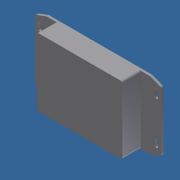
# Autodesk Inventor part: LIDAR PSU
Saved by Autodesk Inventor 2012 (Build 160160000, 160)
## iProperties
Created: 2012-03-25
Part Number: LIDAR PSU
Material: Default
Document SubType Name: Modeling
Designer: Edward
Mass: 374.214 g
Surface Area: 436.694 cm^2
Volume: 324.722 cm^3
Density: 1.15241 g/cm^3
Author: Edward
Autodesk Inventor part; units mm, degrees
ref_plane "YZ Plane" through (0, 0, 0) normal (1, 0, 0) x (0, 1, 0)
ref_plane "XZ Plane" through (0, 0, 0) normal (0, 1, 0) x (-1, 0, 0)
ref_plane "XY Plane" through (0, 0, 0) normal (0, 0, 1) x (1, 0, 0)
sketch "Sketch1" plane through (0, 0, 0) normal (0, 0, 1) x (1, 0, 0)
  line L0 (-7.8312, -44.5359) -> (133.0626, -44.5359)
  line L1 (133.0626, -44.5359) -> (133.0626, 47.9201)
  line L2 (133.0626, 47.9201) -> (-7.8312, 47.9201)
  line L3 (-7.8312, 47.9201) -> (-7.8312, -44.5359)
  line L4 (-7.8312, 47.9201) -> (-21.6516, 42.767)
  arc A0 (-21.6516, 42.767) -> (-23.7173, 39.7921) centre (-20.5423, 39.7921) ccw
  line L5 (-23.7173, 39.7921) -> (-23.7173, -36.4079)
  arc A1 (-23.7173, -36.4079) -> (-21.6516, -39.3828) centre (-20.5423, -36.4079) ccw
  line L6 (-21.6516, -39.3828) -> (-7.8312, -44.5359)
  circle A2 centre (-17.0085, 33.8104) radius 2.1971
  circle A3 centre (-17.0085, 27.689) radius 2.1971
  line L7 (-19.2056, 33.8104) -> (-14.8114, 33.8104)
  line L8 (-14.8114, 33.8104) -> (-14.8114, 27.689)
  line L9 (-14.8114, 27.689) -> (-19.2056, 27.689)
  line L10 (-19.2056, 27.689) -> (-19.2056, 33.8104)
  line L11 (-7.8312, 1.6921) -> (-23.7173, 1.6921)
  circle A4 centre (-17.0085, -30.4262) radius 2.1971
  circle A5 centre (-17.0085, -24.3048) radius 2.1971
  line L12 (-19.2056, -30.4262) -> (-14.8114, -30.4262)
  line L13 (-14.8114, -30.4262) -> (-14.8114, -24.3048)
  line L14 (-14.8114, -24.3048) -> (-19.2056, -24.3048)
  line L15 (-19.2056, -24.3048) -> (-19.2056, -30.4262)
  line L16 (62.6157, 47.9201) -> (62.6157, -44.5359)
  line L17 (133.0626, 47.9201) -> (146.8831, 42.767)
  arc A6 (148.9488, 39.7921) -> (146.8831, 42.767) centre (145.7738, 39.7921) ccw
  line L18 (148.9488, 39.7921) -> (148.9488, -36.4079)
  arc A7 (146.8831, -39.3828) -> (148.9488, -36.4079) centre (145.7738, -36.4079) ccw
  line L19 (146.8831, -39.3828) -> (133.0626, -44.5359)
  circle A8 centre (142.24, 33.8104) radius 2.1971
  circle A9 centre (142.24, 27.689) radius 2.1971
  line L20 (144.4371, 33.8104) -> (140.0429, 33.8104)
  line L21 (140.0429, 33.8104) -> (140.0429, 27.689)
  line L22 (140.0429, 27.689) -> (144.4371, 27.689)
  line L23 (144.4371, 27.689) -> (144.4371, 33.8104)
  line L24 (133.0626, 1.6921) -> (148.9488, 1.6921)
  circle A10 centre (142.24, -30.4262) radius 2.1971
  line L25 (144.4371, -30.4262) -> (140.0429, -30.4262)
  line L26 (140.0429, -30.4262) -> (140.0429, -24.3048)
  line L27 (140.0429, -24.3048) -> (144.4371, -24.3048)
  line L28 (144.4371, -24.3048) -> (144.4371, -30.4262)
  circle A11 centre (142.24, -24.3048) radius 2.1971
  point P0 (0, 0)
  point P1 (125.2315, 0)
  dimension "d4" = 4.3942
  dimension "d0" = 92.456
  dimension "d1" = 140.8938
  dimension "d2" = 3.175
  dimension "d3" = 76.2
  dimension "d5" = 6.1214
  dimension "d6" = 25.9969
  constraints: 58 end point, 27 symmetric about line, 9 horizontal alignment, 8 point on circle, 8 vertical, 5 parallel, 4 centre point, 4 horizontal, 4 midpoint, 3 perpendicular, 3 tangent, 1 equal length, 1 equal radius, 18 other
  measures "d0" distance between parallel lines of L0 L2
  measures "d1" distance of L1.end L2.end
  measures "d2" radius of A0
  measures "d3" distance of L5.start L5.end
  measures "d5" distance between parallel lines of L9 L7
  measures "d6" distance from line of point (-17.008, 27.689) L11
extrude "Extrusion1" add sketch "Sketch1" along normal blind 3.175
sketch "Sketch2" plane through (0, 0, 3.175) normal (0, 0, 1) x (1, 0, 0)
  line L0 (133.0626, -44.5359) -> (-7.8312, -44.5359) projected
  line L1 (-7.8312, 47.9201) -> (133.0626, 47.9201) projected
  line L2 (7.1548, 47.9201) -> (118.0766, 47.9201)
  line L3 (121.2516, 44.7451) -> (121.2516, -41.3609)
  line L4 (118.0766, -44.5359) -> (7.1548, -44.5359)
  line L5 (3.9798, -41.3609) -> (3.9798, 44.7451)
  arc A0 (7.1548, 47.9201) -> (3.9798, 44.7451) centre (7.1548, 44.7451) ccw
  arc A1 (3.9798, -41.3609) -> (7.1548, -44.5359) centre (7.1548, -41.3609) ccw
  arc A2 (118.0766, -44.5359) -> (121.2516, -41.3609) centre (118.0766, -41.3609) ccw
  arc A3 (121.2516, 44.7451) -> (118.0766, 47.9201) centre (118.0766, 44.7451) ccw
  point P0 (0, 0)
  point P1 (3.9798, 47.9201)
  point P2 (121.2516, -44.5359)
  point P3 (62.6157, 47.9201)
  dimension "d9" = 117.2718
  dimension "d10" = 3.175
  constraints: 8 end point, 8 point on circle, 8 tangent, 6 point on line, 4 centre point, 3 equal radius, 2 midpoint, 2 parallel, 1 horizontal, 1 perpendicular
  measures "d9" distance between parallel lines of L5 L3
  measures "d10" radius of A0
extrude "Extrusion2" add sketch "Sketch2" along normal blind 25.4
body "Solid1"
